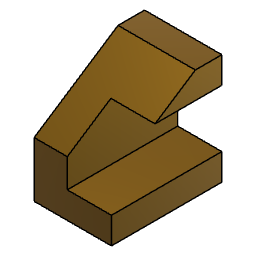
3d15 v1 (Autodesk Fusion 360 design; units mm, degrees)
Autodesk Fusion 360 part; units mm, degrees
sketch "Sketch1" plane through (0, 0, 0) normal (0, 0, 1) x (1, 0, 0)
  line L0 (0, 0) -> (0, 25)
  line L1 (0, 25) -> (15, 25)
  line L2 (15, 25) -> (15, 12)
  line L3 (15, 12) -> (35, 12)
  line L4 (35, 12) -> (35, 0)
  line L5 (35, 0) -> (0, 0)
  dimension "d1" = 25
  dimension "d2" = 20
  dimension "d3" = 35
  dimension "d4" = 12
  constraint coincident L0.start L5.end
  constraint vertical L0
  constraint perpendicular L0 L1
  constraint perpendicular L1 L2
  constraint perpendicular L2 L3
  constraint perpendicular L3 L4
  constraint perpendicular L0 L5
  measures "d1" distance of L0.start L0.end
  measures "d2" distance of L2.end L3.end
  measures "d3" distance of L4.end L0.start
  measures "d4" distance of L3.end L4.end
extrude "Extrude1" add sketch "Sketch1" along normal mid plane 50
sketch "Sketch2" plane through (0, 0, 0) normal (-1, 0, 0) x (0, 0, 1)
  line L0 (-25, 0) -> (25, 0)
  line L1 (25, 0) -> (25, 25)
  line L2 (25, 25) -> (-25, 25)
  line L3 (-25, 25) -> (-25, 0)
  line L4 (-25, 25) -> (-25, 50)
  line L5 (-25, 50) -> (-13, 50)
  line L6 (-13, 50) -> (25, 25)
  dimension "d7" = 25
  dimension "d8" = 12
  constraint coincident L2.end L3.start
  constraint perpendicular L2 L4
  constraint perpendicular L4 L5
  constraint coincident L1.end L2.start
  measures "d7" distance of L2.end L4.end
  measures "d8" distance of L4.end L5.end
extrude "Extrude2" add sketch "Sketch2" against normal blind 15 contours L2 L4 L5 L6
sketch "Sketch3" plane through (15, 0, 0) normal (1, 0, 0) x (0, 0, -1)
  line L0 (-25, 25) -> (-25, 12)
  line L1 (-25, 12) -> (25, 12)
  line L2 (25, 12) -> (25, 50)
  line L3 (25, 50) -> (13, 50)
  line L4 (13, 50) -> (-25, 25)
  line L5 (-5.24, 38) -> (25, 38)
  dimension "d11" = 12
  constraint perpendicular L2 L5
  constraint coincident L4 L5.start
  constraint coincident L2 L5.end
  measures "d11" distance of L3 L5
extrude "Extrude3" add sketch "Sketch3" along normal blind 20 contours L2 L3 L4 L5
